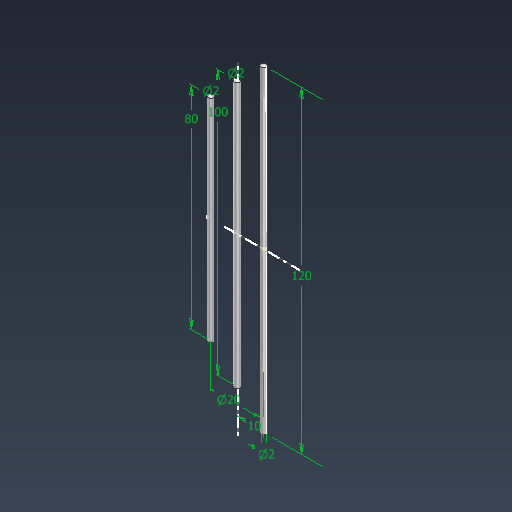
# Autodesk Inventor part: rod
Saved by Autodesk Inventor 2025.3 (Build 293356000, 356)
## iProperties
Created: 2025-09-04
Part Number: rod
Material: 不鏽鋼 AISI 440C、熔接
Document SubType Name: Modeling
Designer: 陳泓任
Density: 7.8 g/cm^3
Appearance: 熔接 - 可鍛鋼
Author: 陳泓任
Autodesk Inventor part; units mm, degrees
ref_plane "YZ Plane" through (0, 0, 0) normal (1, 0, 0) x (0, 1, 0)
ref_plane "XZ Plane" through (0, 0, 0) normal (0, 1, 0) x (-1, 0, 0)
ref_plane "XY Plane" through (0, 0, 0) normal (0, 0, 1) x (1, 0, 0)
sketch "草圖1" plane through (0, 0, 0) normal (0, 0, 1) x (1, 0, 0)
  line L0 (0, 60) -> (1, 60)
  line L1 (1, 60) -> (1, -60)
  line L2 (1, -60) -> (0, -60)
  line L3 (0, -60) -> (0, 60)
  line L4 (0, 49.2923) -> (0, -49.2923)
  line L5 (-11, 50) -> (-10, 50)
  line L6 (-10, 50) -> (-10, -50)
  line L7 (-10, -50) -> (-11, -50)
  line L8 (-11, -50) -> (-11, 50)
  line L9 (-10, 56.3661) -> (-10, -65.7059)
  line L10 (-14.7421, 0) -> (13.3348, 0)
  line L11 (-21, 40) -> (-20, 40)
  line L12 (-20, 40) -> (-20, -40)
  line L13 (-20, -40) -> (-21, -40)
  line L14 (-21, -40) -> (-21, 40)
  point P0 (0, 0)
  point P1 (0, 0)
  point P2 (-11, 0)
  point P3 (-10, 0)
  point P4 (-21, 0)
  dimension "d1" = 120
  dimension "d2" = 2
  dimension "d4" = 10
  dimension "d5" = 2
  dimension "d6" = 100
  dimension "d8" = 80
  dimension "d9" = 20
  dimension "d10" = 2
  constraints: 30 end point, 6 parallel, 5 midpoint, 4 horizontal, 3 perpendicular, 3 point on line, 2 vertical, 1 coincident, 1 collinear
  measures "d1" distance of L0.end L1.end
  measures "d2" diameter of L1 L4
  measures "d4" distance between parallel lines of L9 L4
  measures "d5" diameter of L8 L9
  measures "d6" distance of L7.end L5.start
  measures "d8" distance of L14.start L14.end
  measures "d9" diameter of L12 L9
  measures "d10" diameter of L14 L12
revolve "迴轉1" add sketch "草圖1" angle 360 about axis through (0, 49.2923, 0) along (0, -1, 0) contours L0 L1 L10 L3 | L1 L2 L3 L10
revolve "迴轉2" add sketch "草圖1" angle 360 about axis through (-10, 56.3661, 0) along (0, -1, 0) separate body contours L6 L7 L8 L10 | L10 L8 L5 L6
revolve "迴轉3" add sketch "草圖1" angle 360 about axis through (-20, 40, 0) along (0, -1, 0) separate body contours L11 L12 L13 L14
